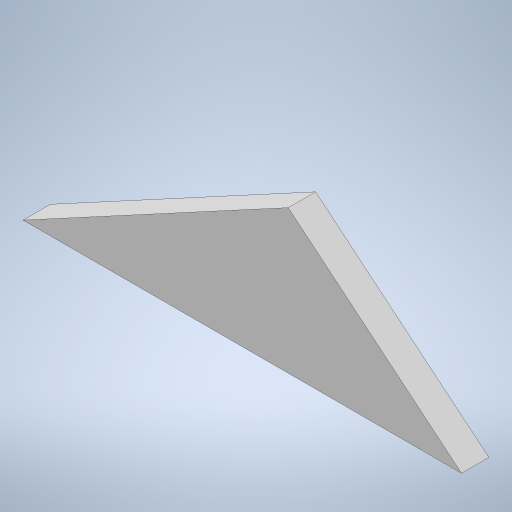
# Autodesk Inventor part: flap
Saved by Autodesk Inventor 2023 (Build 270158000, 158)
## iProperties
Created: 2024-02-01
Part Number: flap
Material: Ogólny
Document SubType Name: Modeling
Designer: domin
Density: 1 g/cm^3
Appearance: Domyślna
Author: domin
Autodesk Inventor part; units mm, degrees
ref_plane "YZ Plane" through (0, 0, 0) normal (1, 0, 0) x (0, 1, 0)
ref_plane "XZ Plane" through (0, 0, 0) normal (0, 1, 0) x (-1, 0, 0)
ref_plane "XY Plane" through (0, 0, 0) normal (0, 0, 1) x (1, 0, 0)
sketch "Szkic1" plane through (0, 0, 0) normal (0, 0, 1) x (1, 0, 0)
  line L0 (0, 0) -> (80, 0)
  line L1 (0, 0) -> (48.3834, 26.1543)
  line L2 (48.3834, 26.1543) -> (80, 0)
  dimension "d0" = 80
  dimension "d1" = 55
  dimension "d5" = 39.599
  constraints: 6 end point, 1 horizontal
  measures "d0" distance of L0.start L0.end
  measures "d1" distance of L0.start L1.end
  measures "d5" angle of L2 L0
extrude "Wyciągnięcie proste1" add sketch "Szkic1" along normal blind 5
